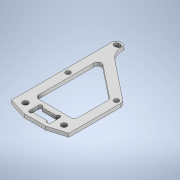
# Autodesk Inventor part: UpperArm_side_frame
Saved by Autodesk Inventor 2020.4 (Build 244396000, 396)
## iProperties
Created: 2021-09-30
Part Number: UpperArm_side_frame
Material: GFRP
Document SubType Name: Modeling
Designer: naoki
Density: 1.75 g/cm^3
Appearance: 滑らか - 淡い灰色
Author: naoki
Comments: GFRP T2
Autodesk Inventor part; units mm, degrees
ref_plane "YZ Plane" through (0, 0, 0) normal (1, 0, 0) x (0, 1, 0)
ref_plane "XZ Plane" through (0, 0, 0) normal (0, 1, 0) x (-1, 0, 0)
ref_plane "XY Plane" through (0, 0, 0) normal (0, 0, 1) x (1, 0, 0)
sketch "スケッチ1" plane through (0, 0, 0) normal (0, 1, 0) x (-1, 0, 0)
  line L0 (-16, 21.5) -> (16, 21.5) construction
  line L1 (16, 21.5) -> (16, -21.5) construction
  line L2 (16, -21.5) -> (-16, -21.5) construction
  line L3 (-16, -21.5) -> (-16, 21.5) construction
  line L4 (-16, 21.5) -> (16, -21.5) construction
  line L5 (16, 21.5) -> (-16, -21.5) construction
  line L6 (0, -35.1049) -> (0, 50.5) construction
  line L7 (34.5893, 0) -> (-34.3502, 0) construction
  circle A0 centre (0, -9.5) radius 10.5 construction
  arc A1 (-16, -9.5) -> (-10.5361, -21.5412) centre (0, -9.5) ccw construction
  arc A2 (10.5361, -21.5412) -> (16, -9.5) centre (0, -9.5) ccw construction
  circle A3 centre (-13.5, -8.5) radius 1.3 construction
  circle A4 centre (-13.5, 18.5) radius 1.3 construction
  circle A5 centre (13.5, -8.5) radius 1.3 construction
  circle A6 centre (13.5, 18.5) radius 1.3 construction
  line L8 (-16, 18.5) -> (-16, 50.5)
  line L9 (16, 18.5) -> (16, 50.5)
  line L10 (16, 50.5) -> (-16, 50.5) construction
  line L11 (6, 42.5) -> (0, 42.5) construction
  line L12 (16, 47.5) -> (6, 47.5) construction
  line L13 (-16, 47.5) -> (-6, 50.5)
  line L14 (6, 50.5) -> (-6, 50.5)
  circle A7 centre (-10.75, 45) radius 1.55
  circle A8 centre (10.75, 45) radius 1.55
  circle A9 centre (0, -9.5) radius 11
  line L15 (13.5, -8.5) -> (12.5, -8.5) construction
  line L16 (13.5, -7.15) -> (12.5, -7.15)
  line L17 (12.5, -9.85) -> (13.5, -9.85)
  arc A10 (13.5, -9.85) -> (13.5, -7.15) centre (13.5, -8.5) ccw
  arc A11 (12.5, -7.15) -> (12.5, -9.85) centre (12.5, -8.5) ccw
  line L18 (-13.5, -8.5) -> (-12.5, -8.5) construction
  line L19 (-13.5, -7.15) -> (-12.5, -7.15)
  line L20 (-12.5, -9.85) -> (-13.5, -9.85)
  arc A12 (-13.5, -7.15) -> (-13.5, -9.85) centre (-13.5, -8.5) ccw
  arc A13 (-12.5, -9.85) -> (-12.5, -7.15) centre (-12.5, -8.5) ccw
  arc A14 (-15.0569, 16.544) -> (-16, 18.5) centre (-13.5, 18.5) ccw construction
  arc A15 (-16, 18.5) -> (-15.0569, 16.544) centre (-13.5, 18.5) ccw
  line L21 (13.5, -6) -> (12.5, -6) construction
  arc A16 (12.5, -6) -> (12.5, -11) centre (12.5, -8.5) ccw construction
  line L22 (12.5, -11) -> (13.5, -11) construction
  arc A17 (13.5, -11) -> (13.5, -6) centre (13.5, -8.5) ccw construction
  line L23 (16, 18.5) -> (16, -8.5)
  arc A18 (13.5, -11) -> (16, -8.5) centre (13.5, -8.5) ccw
  arc A19 (10.9574, -10.4673) -> (12.5, -11) centre (12.5, -8.5) ccw
  line L24 (13.5, -11) -> (12.5, -11)
  circle A20 centre (-13.5, 18.5) radius 1.35
  circle A21 centre (13.5, 18.5) radius 1.35
  line L25 (-15.0569, 16.544) -> (6.8505, -0.8935)
  line L26 (16, 42.5) -> (6, 42.5) construction
  line L27 (11, 39.5) -> (-11, 39.5)
  line L28 (11, 2.1941) -> (11, 39.5)
  line L29 (11, 2.1941) -> (-11, 19.7054)
  line L30 (-11, 19.7054) -> (-11, 39.5)
  line L31 (6, 42.5) -> (-6, 42.5) construction
  line L32 (6, 47.5) -> (-16, 47.5) construction
  line L33 (-6, 42.5) -> (-16, 42.5) construction
  line L34 (-6, 47.5) -> (6, 47.5) construction
  line L35 (6, 47.5) -> (6, 42.5) construction
  line L36 (6, 42.5) -> (-6, 42.5) construction
  line L37 (-6, 42.5) -> (-6, 47.5) construction
  line L38 (-6, 47.5) -> (6, 42.5) construction
  line L39 (6, 47.5) -> (-6, 42.5) construction
  line L40 (16, 47.5) -> (6, 50.5)
  line L41 (6, 42.5) -> (-6, 42.5) construction
  line L42 (-6, 42.5) -> (-6, 47.5) construction
  line L43 (-6, 47.5) -> (6, 47.5) construction
  line L44 (6, 47.5) -> (6, 42.5) construction
  line L45 (6.01, 42.49) -> (-6.01, 42.49)
  line L46 (-6.01, 42.49) -> (-6.01, 47.51)
  line L47 (-6.01, 47.51) -> (6.01, 47.51)
  line L48 (6.01, 47.51) -> (6.01, 42.49)
  line L49 (6.01, 45) -> (-6.01, 45) construction
  arc A22 (-6.01, 42.49) -> (-3.91, 42.5) centre (-4.96, 42.49) ccw
  line L50 (0, 125.1049) -> (0, 39.5) construction
  arc A23 (-3.91, 47.5) -> (-6.01, 47.51) centre (-4.96, 47.51) ccw
  arc A24 (3.91, 42.5) -> (6.01, 42.49) centre (4.96, 42.49) ccw
  arc A25 (6.01, 47.51) -> (3.91, 47.5) centre (4.96, 47.51) ccw
  point P0 (0, 0)
  point P1 (0, 0)
  point P2 (0, 0)
  point P3 (13, -8.5)
  point P4 (-13, -8.5)
  point P5 (0, 45)
  point P6 (0, 45)
  point P7 (3.91, 42.49)
  point P8 (-3.91, 42.49)
  point P9 (-3.91, 47.51)
  point P10 (3.91, 47.51)
  dimension "d0" = 32
  dimension "d1" = 43
  dimension "d2" = 9.5
  dimension "d3" = 8.5
  dimension "d4" = 18.5
  dimension "d5" = 13.5
  dimension "d6" = 13.5
  dimension "d7" = 21
  dimension "d8" = 16
  dimension "d9" = 2.6
  dimension "d10" = 2.6
  dimension "d17" = 32
  dimension "d18" = 32
  dimension "d26" = 3.1
  dimension "d28" = 1
  dimension "d29" = 2.7
  dimension "d30" = 22
  dimension "d31" = 2.7
  dimension "d32" = 3
  dimension "d33" = 5
  dimension "d34" = 5
  dimension "d35" = 5
  dimension "d36" = 3
  dimension "d37" = 5
  dimension "d38" = 10
  dimension "d39" = 10
  dimension "d40" = 3
  dimension "d41" = 10
  dimension "d42" = 0.01
  dimension "d43" = 1.05
  dimension "d48" = 21.5
  constraints: 106 end point, 36 point on circle, 26 centre point, 25 symmetric about line, 20 point on line, 14 parallel, 12 midpoint, 11 perpendicular, 8 coincident, 8 tangent, 6 horizontal, 3 horizontal alignment, 2 collinear, 2 concentric, 1 vertical, 16 other
  measures "d0" distance of L1.end L2.end
  measures "d1" distance of L0.end L1.end
  measures "d2" distance of point (0, 0) point (0, -9.5)
  measures "d3" distance from line of point (-13.5, -8.5) L7
  measures "d4" distance from line of L7 point (-13.5, 18.5)
  measures "d5" distance from line of L6 point (-13.5, -8.5)
  measures "d6" distance from line of L6 point (-13.5, 18.5)
  measures "d7" diameter of A0
  measures "d8" radius of A1
  measures "d9" diameter of A3
  measures "d10" diameter of A4
  measures "d17" distance of L8.start L8.end
  measures "d18" distance of L9.start L9.end
  measures "d26" diameter of A7
  measures "d28" distance of L15.start L15.end
  measures "d29" diameter of A11
  measures "d30" diameter of A9
  measures "d31" diameter of A20
  measures "d32" distance between parallel lines of L26 L27
  measures "d33" distance between parallel lines of L25 L29
  measures "d34" distance between parallel lines of L8 L30
  measures "d35" distance between parallel lines of L28 L9
  measures "d36" distance between parallel lines of L14 L34
  measures "d37" distance of L36.end L34.start
  measures "d38" distance between parallel lines of L8 L37
  measures "d39" distance from line of L8 L13.end
  measures "d40" distance from line of L10 L13.start
  measures "d41" distance from line of L9 L14.start
  measures "d42" distance between parallel lines of L36 L45
  measures "d43" distance from line of L46 point (-4.96, 42.49)
  measures "d48" distance of A7.centre A8.centre
extrude "押し出し1" add sketch "スケッチ1" along normal blind 2 contours L8 L13 L14 L40 L9 L23 A18 L24 A19 A9 L25 A15
fillet "フィレット1" radius 2.1 4 edges at (-11, 1, 2.1941) (11, 1, 39.5) (-11, 1, 39.5) (11, 1, 19.7054)
fillet "フィレット2" radius 1 1 edges at (-10.9574, 1, -10.4673)
equation "\"d6\" = d5"
equation "\"d18\" = d17"
